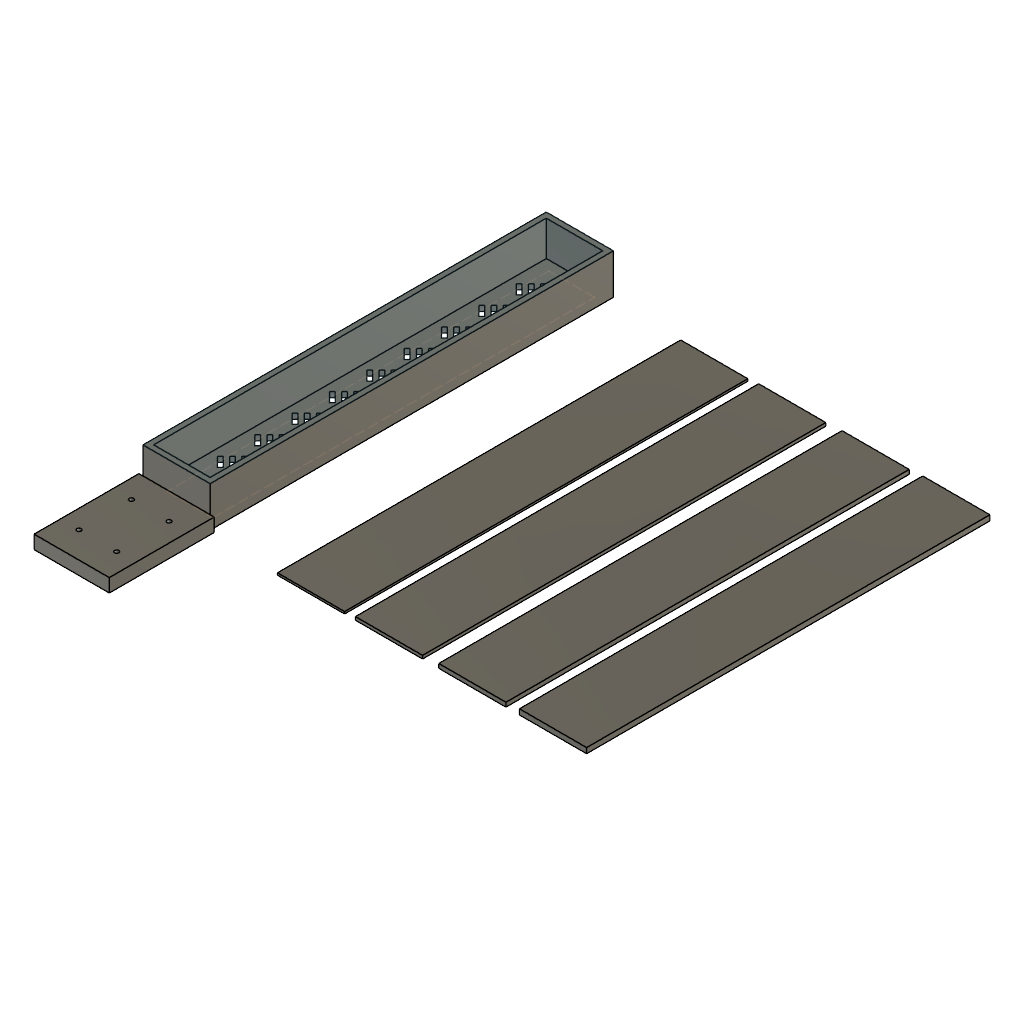
blade_lamp (Autodesk Fusion 360 design; units mm, degrees)
Autodesk Fusion 360 part; units mm, degrees
sketch "Sketch1" plane through (0, 0, 0) normal (0, 0, 1) x (1, 0, 0)
  line L0 (0, 0) -> (25, 0)
  line L1 (25, 0) -> (25, 150)
  line L2 (25, 150) -> (0, 150)
  line L3 (0, 150) -> (0, 0)
  dimension "d1" = 25
  dimension "d2" = 150
  constraint horizontal L0
  constraint vertical L1
  constraint horizontal L2
  constraint vertical L3
  constraint coincident L0.start L3.end
  measures "d1" distance of L0.start L0.end
  measures "d2" distance of L0.start L2.end
extrude "Extrude1" add sketch "Sketch1" along normal blind 15 makes body 1
shell "Shell1" thickness 2 removed faces 1 at (8.3333, 100, 15) on bodies 1
sketch "Sketch4" plane through (0, 0, 2) normal (0, 0, 1) x (-1, 0, 0)
  line L0 (-2, -148) -> (-2, -2)
  line L1 (-2, -2) -> (-23, -2)
  line L2 (-23, -2) -> (-23, -148)
  line L3 (-23, -148) -> (-2, -148)
  line L4 (1.5, 0) -> (-26.5, 0)
  line L5 (-26.5, 0) -> (-26.5, 39)
  line L6 (-26.5, 39) -> (1.5, 39)
  line L7 (1.5, 39) -> (1.5, 0)
  dimension "d8" = 28
  dimension "d9" = 39
  dimension "d10" = 1.5
  constraint horizontal L4
  constraint vertical L5
  constraint horizontal L6
  constraint vertical L7
  measures "d8" distance of L4.start L4.end
  measures "d9" distance of L4.start L6.end
  measures "d10" distance of origin L4.start
move_body "Move1" bodies 1 to x (1, 0, 0) y (0, 1, 0) z (0, 0, 1) at (0, 0, 2)
extrude "Extrude2" add sketch "Sketch4" along normal blind 3 contours L4 L5 L6 L7 bodies 1
sketch "Sketch5" plane through (0, 0, 0) normal (0, 0, 1) x (1, 0, 0)
  line L0 (21, 147, 1.5) -> (4, 147, 1.5) construction
  line L1 (4, 147, 1.5) -> (4, 5, 1.5) construction
  line L2 (4, 5, 1.5) -> (21, 5, 1.5) construction
  line L3 (21, 5, 1.5) -> (21, 147, 1.5) construction
  dimension "d22" = 17
  dimension "d23" = 142
sketch "Sketch6" plane through (0, 0, 0) normal (0, 0, 1) x (1, 0, 0)
  line L0 (16.9248, 146.6721, 1.5021) -> (15.8641, 145.6114, 1.5021)
  line L1 (15.8641, 145.6114, 1.5021) -> (19.3997, 142.0759, 1.5021)
  line L2 (19.3997, 142.0759, 1.5021) -> (20.4603, 143.1366, 1.5021)
  line L3 (20.4603, 143.1366, 1.5021) -> (16.9248, 146.6721, 1.5021)
  dimension "d29" = 1.5
  dimension "d30" = 5
extrude "Extrude3" cut sketch "Sketch6" along normal mid plane 6 contours L0 L1 L2 L3 in plane through (0, 0, 1.5021) normal (0, 0, 1) bodies 1
pattern_linear "R-Pattern1" count 1 spacing 0 along (-0.707107, 0.707107, 0) count 6 spacing 3.2 along (-0.707107, -0.707107, 0) of "Extrude3"
pattern_linear "R-Pattern2" count 10 spacing 13.8889 along (0, -1, 0) of "Extrude3", "R-Pattern1"
extrude "Extrude4" add 1 faces at (16.6667, -26, 5) along direction (0, 0, 1) blind 2 on bodies 1 bodies 1
sketch "Sketch7" plane through (0, 0, 17) normal (0, 0, 1) x (-1, 0, 0)
  line L0 (-2, -148) -> (-23, -148)
  line L1 (-23, -148) -> (-23, -2)
  line L2 (-23, -2) -> (-2, -2)
  line L3 (-2, -2) -> (-2, -148)
  line L4 (0, -150) -> (0, 0)
  line L5 (0, 0) -> (-25, 0)
  line L6 (-25, 0) -> (-25, -150)
  line L7 (-25, -150) -> (0, -150)
sketch "Sketch8" plane through (0, 0, 7) normal (0, 0, 1) x (-1, 0, 0)
hole "Hole5" at (5.5, -29.25, 7) direction (0, 0, -1) diameter 1.6 end through all bodies 1
hole "Hole6" at (19.5204, -29.2643, 7) direction (0, 0, -1) diameter 1.6 end through all bodies 1
hole "Hole7" at (5.5, -9.75, 7) direction (0, 0, -1) diameter 1.6 end through all bodies 1
hole "Hole8" at (19.4998, -9.7495, 7) direction (0, 0, -1) diameter 1.6 end through all bodies 1
sketch "Sketch9" plane through (0, 0, 0) normal (0, 0, 1) x (1, 0, 0)
  line L0 (50, 150) -> (75, 150)
  line L1 (75, 150) -> (75, 0)
  line L2 (75, 0) -> (50, 0)
  line L3 (50, 0) -> (50, 150)
  dimension "d51" = 25
  dimension "d52" = 150
  constraint horizontal L0
  constraint vertical L1
  constraint horizontal L2
  constraint vertical L3
  measures "d51" distance of L0.start L0.end
  measures "d52" distance of L0.start L2.end
hole "Hole9" at (12.635, 8.0234, 4) direction (0, 0, -1) diameter 10 end through all bodies 1
extrude "Extrude5" add sketch "Sketch9" along normal blind 0.8 separate body makes body 2
copy_body "CopyPasteBodies1" bodies 2 makes body 3
move_body "Move2" bodies 3 to x (1, 0, 0) y (0, 1, 0) z (0, 0, 1) at (29, 0, 0)
extrude "Extrude6" add 1 faces at (87.3333, 100, 0.8) along direction (0, 0, 1) blind 0.4 on bodies 3 bodies 3
copy_body "CopyPasteBodies2" bodies 3 makes body 4
move_body "Move3" bodies 4 to x (1, 0, 0) y (0, 1, 0) z (0, 0, 1) at (31, 0, 0)
extrude "Extrude7" add 1 faces at (118.3333, 100, 1.2) along direction (0, 0, 1) blind 0.4 on bodies 4 bodies 4
copy_body "CopyPasteBodies3" bodies 4 makes body 5
move_body "Move4" bodies 5 to x (1, 0, 0) y (0, 1, 0) z (0, 0, 1) at (30, 0, 0)
extrude "Extrude8" add 1 faces at (148.3333, 100, 1.6) along direction (0, 0, 1) blind 1.2 on bodies 5 bodies 5
extrude "Extrude9" cut 1 faces at (148.3333, 100, 2.8) along direction (0, 0, 1) mid plane 1.6 on bodies 5 bodies 5
